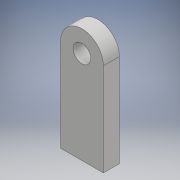
# Autodesk Inventor part: Part2
Saved by Autodesk Inventor 2018 (Build 220112000, 112)
## iProperties
Created: 2018-02-02
Part Number: Part2
Material: Generic
Document SubType Name: Modeling
Designer: eroldan
Density: 1 g/cm^3
Appearance: Default
Author: eroldan
Autodesk Inventor part; units mm, degrees
ref_plane "YZ Plane" through (0, 0, 0) normal (1, 0, 0) x (0, 1, 0)
ref_plane "XZ Plane" through (0, 0, 0) normal (0, 1, 0) x (-1, 0, 0)
ref_plane "XY Plane" through (0, 0, 0) normal (0, 0, 1) x (1, 0, 0)
sketch "Sketch1" plane through (0, 0, 0) normal (0, 1, 0) x (-1, 0, 0)
  line L0 (4, 0) -> (-4, 0)
  line L1 (4, 0) -> (4, 12)
  line L2 (-4, 0) -> (-4, 12)
  arc A0 (4, 17.3329) -> (-4, 17.3329) centre (0, 17.3329) ccw
  line L3 (4, 17.3329) -> (4, 12)
  line L4 (-4, 17.3329) -> (-4, 12)
  circle A1 centre (0, 17.3329) radius 1.65
  point P0 (0, 0)
  point P1 (0, 0)
  dimension "d0" = 8
  dimension "d1" = 12
  dimension "d9" = 8
  dimension "d12" = 3.3
  constraints: 10 end point, 2 centre point, 2 coincident, 2 point on circle, 2 tangent, 2 vertical, 1 horizontal, 1 horizontal alignment, 1 midpoint, 1 vertical alignment
  measures "d0" distance of L0.start L0.end
  measures "d1" distance of L0.start L1.end
  measures "d9" distance of L4.start L3.start
  measures "d12" diameter of A1
extrude "Extrusion1" add sketch "Sketch1" along normal blind 3
body "Solid1"
